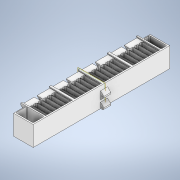
# Autodesk Inventor part: cajas_V2
Saved by Autodesk Inventor 2020.3 (Build 243373000, 373)
## iProperties
Created: 2021-02-18
Part Number: cajas_V2
Material: PET Plastic
Document SubType Name: Modeling
Designer: juanp
Density: 1.541 g/cm^3
Appearance: Polycarbonate - Clear
Author: juanp
Autodesk Inventor part; units mm, degrees
ref_plane "YZ Plane" through (0, 0, 0) normal (1, 0, 0) x (0, 1, 0)
ref_plane "XZ Plane" through (0, 0, 0) normal (0, 1, 0) x (-1, 0, 0)
ref_plane "XY Plane" through (0, 0, 0) normal (0, 0, 1) x (1, 0, 0)
sketch "Sketch1" plane through (0, 0, 0) normal (0, 1, 0) x (-1, 0, 0)
  line L0 (0, 0) -> (56, 0) construction
  line L1 (56, 0) -> (56, -330)
  line L2 (0, -330) -> (0, 0)
  line L3 (54, -4) -> (4, -4) construction
  line L4 (4, -4) -> (4, -15.1667)
  line L5 (4, -15.1667) -> (54, -15.1667)
  line L6 (54, -15.1667) -> (54, -4)
  line L7 (54, -19.1667) -> (4, -19.1667)
  line L8 (4, -19.1667) -> (4, -30.3333)
  line L9 (4, -30.3333) -> (54, -30.3333)
  line L10 (54, -30.3333) -> (54, -19.1667)
  line L11 (54, -32.3333) -> (4, -32.3333)
  line L12 (4, -32.3333) -> (4, -43.5)
  line L13 (4, -43.5) -> (54, -43.5)
  line L14 (54, -43.5) -> (54, -32.3333)
  line L15 (54, -45.5) -> (4, -45.5)
  line L16 (4, -45.5) -> (4, -56.6667)
  line L17 (4, -56.6667) -> (54, -56.6667)
  line L18 (54, -56.6667) -> (54, -45.5)
  line L19 (54, -58.6667) -> (4, -58.6667)
  line L20 (4, -58.6667) -> (4, -69.8333)
  line L21 (4, -69.8333) -> (54, -69.8333)
  line L22 (54, -69.8333) -> (54, -58.6667)
  line L23 (54, -71.8333) -> (4, -71.8333)
  line L24 (4, -71.8333) -> (4, -83)
  line L25 (4, -83) -> (54, -83)
  line L26 (54, -83) -> (54, -71.8333)
  line L27 (54, -85) -> (4, -85)
  line L28 (4, -85) -> (4, -96.1667)
  line L29 (4, -96.1667) -> (54, -96.1667)
  line L30 (54, -96.1667) -> (54, -85)
  line L31 (54, -102.1667) -> (4, -102.1667)
  line L32 (4, -102.1667) -> (4, -113.3333)
  line L33 (4, -113.3333) -> (54, -113.3333)
  line L34 (54, -113.3333) -> (54, -102.1667)
  line L35 (54, -115.3333) -> (4, -115.3333)
  line L36 (4, -115.3333) -> (4, -126.5)
  line L37 (4, -126.5) -> (54, -126.5)
  line L38 (54, -126.5) -> (54, -115.3333)
  line L39 (54, -128.5) -> (4, -128.5)
  line L40 (4, -128.5) -> (4, -139.6667)
  line L41 (4, -139.6667) -> (54, -139.6667)
  line L42 (54, -139.6667) -> (54, -128.5)
  line L43 (54, -141.6667) -> (4, -141.6667)
  line L44 (4, -141.6667) -> (4, -152.8333)
  line L45 (4, -152.8333) -> (54, -152.8333)
  line L46 (54, -152.8333) -> (54, -141.6667)
  line L47 (54, -154.8333) -> (4, -154.8333)
  line L48 (4, -154.8333) -> (4, -166)
  line L49 (4, -166) -> (54, -166)
  line L50 (54, -166) -> (54, -154.8333)
  line L51 (54, -168) -> (4, -168)
  line L52 (4, -168) -> (4, -179.1667)
  line L53 (4, -179.1667) -> (54, -179.1667)
  line L54 (54, -179.1667) -> (54, -168)
  line L55 (54, -185.1667) -> (4, -185.1667)
  line L56 (4, -185.1667) -> (4, -196.3333)
  line L57 (4, -196.3333) -> (54, -196.3333)
  line L58 (54, -196.3333) -> (54, -185.1667)
  line L59 (54, -198.3333) -> (4, -198.3333)
  line L60 (4, -198.3333) -> (4, -209.5)
  line L61 (4, -209.5) -> (54, -209.5)
  line L62 (54, -209.5) -> (54, -198.3333)
  line L63 (54, -211.5) -> (4, -211.5)
  line L64 (4, -211.5) -> (4, -222.6667)
  line L65 (4, -222.6667) -> (54, -222.6667)
  line L66 (54, -222.6667) -> (54, -211.5)
  line L67 (54, -224.6667) -> (4, -224.6667)
  line L68 (4, -224.6667) -> (4, -235.8333)
  line L69 (4, -235.8333) -> (54, -235.8333)
  line L70 (54, -235.8333) -> (54, -224.6667)
  line L71 (56, -330) -> (56, -349.1667)
  line L72 (56, -349.1667) -> (0, -349.1667) construction
  line L73 (0, -349.1667) -> (0, -330)
  line L74 (54, -237.8333) -> (4, -237.8333)
  line L75 (4, -237.8333) -> (4, -249)
  line L76 (4, -249) -> (54, -249)
  line L77 (54, -249) -> (54, -237.8333)
  line L78 (54, -251) -> (4, -251)
  line L79 (4, -251) -> (4, -262.1667)
  line L80 (4, -262.1667) -> (54, -262.1667)
  line L81 (54, -262.1667) -> (54, -251)
  line L82 (54, -268.1667) -> (4, -268.1667)
  line L83 (4, -268.1667) -> (4, -279.3333)
  line L84 (4, -279.3333) -> (54, -279.3333)
  line L85 (54, -279.3333) -> (54, -268.1667)
  line L86 (54, -281.3333) -> (4, -281.3333)
  line L87 (4, -281.3333) -> (4, -292.5)
  line L88 (4, -292.5) -> (54, -292.5)
  line L89 (54, -292.5) -> (54, -281.3333)
  line L90 (54, -294.5) -> (4, -294.5)
  line L91 (4, -294.5) -> (4, -305.6667)
  line L92 (4, -305.6667) -> (54, -305.6667)
  line L93 (54, -305.6667) -> (54, -294.5)
  line L94 (54, -307.6667) -> (4, -307.6667)
  line L95 (4, -307.6667) -> (4, -318.8333)
  line L96 (4, -318.8333) -> (54, -318.8333)
  line L97 (54, -318.8333) -> (54, -307.6667)
  line L98 (54, -320.8333) -> (4, -320.8333)
  line L99 (4, -320.8333) -> (4, -332)
  line L100 (4, -332) -> (54, -332)
  line L101 (54, -332) -> (54, -320.8333)
  line L102 (54, -334) -> (4, -334)
  line L103 (4, -334) -> (4, -345.1667)
  line L104 (4, -345.1667) -> (54, -345.1667)
  line L105 (54, -345.1667) -> (54, -334)
  line L106 (54, -4) -> (54, 16.4167)
  line L107 (54, 16.4167) -> (4, 16.4167)
  line L108 (4, 16.4167) -> (4, -4)
  line L109 (56, 0) -> (56, 20.4167)
  line L110 (56, 20.4167) -> (0, 20.4167)
  line L111 (0, 20.4167) -> (0, 0)
  line L112 (0, -349.1667) -> (0, -369.5833)
  line L113 (0, -369.5833) -> (56, -369.5833)
  line L114 (56, -369.5833) -> (56, -349.1667)
  line L115 (54, -339.5833) -> (104.9487, -339.5833) construction
  line L116 (104.9487, -339.5833) -> (104.9487, -9.5833) construction
  line L117 (104.9487, -9.5833) -> (54, -9.5833) construction
  line L118 (4, -349.1667) -> (54, -349.1667)
  line L119 (54, -349.1667) -> (54, -365.5833)
  line L120 (54, -365.5833) -> (4, -365.5833)
  line L121 (4, -365.5833) -> (4, -349.1667)
  point P0 (104.9487, -174.5833)
  dimension "d2" = 2
  dimension "d3" = 4
  dimension "d4" = 4
  dimension "d5" = 50
  dimension "d6" = 4
  dimension "d7" = 2
  dimension "d8" = 2
  dimension "d9" = 2
  dimension "d10" = 2
  dimension "d11" = 2
  dimension "d12" = 6
  dimension "d13" = 2
  dimension "d14" = 2
  dimension "d15" = 2
  dimension "d16" = 2
  dimension "d17" = 2
  dimension "d18" = 6
  dimension "d19" = 2
  dimension "d20" = 2
  dimension "d21" = 2
  dimension "d24" = 11.1667
  dimension "d35" = 2
  dimension "d36" = 2
  dimension "d37" = 6
  dimension "d38" = 2
  dimension "d39" = 2
  dimension "d40" = 2
  dimension "d41" = 2
  dimension "d42" = 2
  dimension "d59" = 4
  dimension "d60" = 330
  dimension "d212" = 4
  dimension "d332" = 195
  dimension "d333" = 195
  dimension "d334" = 4
  constraints: 244 end point, 53 parallel, 37 perpendicular, 34 equal length, 33 point on line, 28 horizontal, 8 collinear, 5 vertical, 3 midpoint
  measures "d2" distance between parallel lines of L1 L6
  measures "d3" distance between parallel lines of L0 L3
  measures "d4" distance between parallel lines of L4 L2
  measures "d5" distance of L3.start L3.end
  measures "d6" distance between parallel lines of L7 L5
  measures "d7" distance between parallel lines of L11 L9
  measures "d8" distance between parallel lines of L15 L13
  measures "d9" distance between parallel lines of L19 L17
  measures "d10" distance between parallel lines of L21 L23
  measures "d11" distance between parallel lines of L27 L25
  measures "d12" distance between parallel lines of L31 L29
  measures "d13" distance between parallel lines of L35 L33
  measures "d14" distance between parallel lines of L39 L37
  measures "d15" distance between parallel lines of L43 L41
  measures "d16" distance between parallel lines of L47 L45
  measures "d17" distance between parallel lines of L51 L49
  measures "d18" distance between parallel lines of L55 L53
  measures "d19" distance between parallel lines of L59 L57
  measures "d20" distance between parallel lines of L63 L61
  measures "d21" distance between parallel lines of L67 L65
  measures "d24" distance of L61.end L59.start
  measures "d35" distance between parallel lines of L69 L74
  measures "d36" distance between parallel lines of L78 L76
  measures "d37" distance between parallel lines of L82 L80
  measures "d38" distance between parallel lines of L86 L84
  measures "d39" distance between parallel lines of L90 L88
  measures "d40" distance between parallel lines of L94 L92
  measures "d41" distance between parallel lines of L98 L96
  measures "d42" distance between parallel lines of L102 L100
  measures "d59" distance between parallel lines of L72 L104
  measures "d60" distance of L117.end L115.start
  measures "d212" distance between parallel lines of L107 L110
  measures "d332" distance from line of L110 point (104.949, -174.583)
  measures "d333" distance from line of L113 point (104.949, -174.583)
  measures "d334" distance between parallel lines of L113 L120
extrude "Extrusion1" add sketch "Sketch1" along normal blind 50
sketch "Sketch3" plane through (0, 0, 0) normal (0, -1, 0) x (1, 0, 0)
  line L0 (-56, -369.5833) -> (-56, 20.4167) projected
  line L1 (0, 20.4167) -> (0, -369.5833) projected
  line L2 (-56, 20.4167) -> (0, 20.4167) projected
  line L3 (0, -369.5833) -> (-56, -369.5833) projected
extrude "Extrusion3" add sketch "Sketch3" along normal blind 2
chamfer "Chamfer4" distance 2 angle 45 208 edges at (-54, 25, -128.5) (-4, 25, -126.5) (-54, 25, -141.6667) (-54, 25, -179.1667) (-54, 25, -185.1667) (-4, 25, -141.6667) (-4, 25, -139.6667) (-54, 25, -115.3333) (-4, 25, -115.3333) (-4, 25, -345.1667) (-54, 25, -345.1667) (-4, 25, -128.5) (-4, 25, -332) (-4, 25, -334) (-54, 25, -334) (-54, 25, -332) (-4, 25, -320.8333) (-54, 25, -318.8333) (-4, 25, -318.8333) (-54, 25, -320.8333) (-4, 25, -307.6667) (-54, 25, -305.6667) (-54, 25, -307.6667) (-4, 25, -305.6667) (-4, 25, -294.5) (-54, 25, -292.5) (-4, 25, -292.5) (-54, 25, -294.5) (-4, 25, -281.3333) (-4, 25, -268.1667) (-54, 25, -279.3333) (-4, 25, -279.3333) (-54, 25, -281.3333) (-4, 25, -166) (-4, 25, -168) (-4, 25, -179.1667) (-4, 25, -196.3333) (-4, 25, -185.1667) (-4, 25, -209.5) (-4, 25, -198.3333) (-54, 0, -173.5833) (-4, 0, -173.5833) (-29, 0, -179.1667) (-29, 0, -185.1667) (-54, 0, -190.75) (-4, 0, -190.75) (-4, 0, -203.9167) (-29, 0, -198.3333) (-54, 0, -203.9167) (-29, 0, -196.3333) (-54, 0, -217.0833) (-4, 0, -217.0833) (-29, 0, -222.6667) (-29, 0, -209.5) (-54, 25, -196.3333) (-54, 25, -198.3333) (-54, 25, -209.5) (-4, 25, -211.5) (-54, 25, -211.5) (-54, 25, -222.6667) (-4, 25, -222.6667) (-4, 25, -224.6667) (-54, 25, -224.6667) (-4, 25, -251) (-54, 25, -249) (-4, 25, -249) (-54, 25, -251) (-4, 25, -262.1667) (-54, 25, -262.1667) (-54, 25, -268.1667) (-29, 0, -211.5) (-29, 0, -224.6667) (-54, 0, -230.25) (-4, 0, -230.25) (-29, 0, -235.8333) (-29, 0, -237.8333) (-54, 0, -243.4167) (-4, 0, -243.4167) (-29, 0, -249) (-29, 0, -251) (-54, 0, -256.5833) (-29, 0, -262.1667) (-29, 0, -268.1667) (-54, 0, -273.75) (-29, 0, -279.3333) (-4, 0, -273.75) (-54, 0, -286.9167) (-29, 0, -292.5) (-4, 0, -256.5833) (-29, 0, -281.3333) (-4, 0, -286.9167) (-29, 0, -294.5) (-54, 0, -300.0833) (-4, 0, -300.0833) (-29, 0, -305.6667) (-29, 0, -307.6667) (-54, 0, -313.25) (-4, 0, -313.25) (-29, 0, -318.8333) (-29, 0, -320.8333) (-29, 0, -332) (-4, 0, -326.4167) (-29, 0, -334) (-4, 0, -339.5833) (-29, 0, -345.1667) (-54, 0, -339.5833) (-54, 0, -326.4167) (-4, 25, -237.8333) (-4, 25, -235.8333) (-54, 25, -235.8333) (-54, 25, -237.8333) (-54, 25, -126.5) (-54, 25, -113.3333) (-4, 25, -113.3333) (-4, 25, -102.1667) (-54, 25, -102.1667) (-54, 25, -96.1667) (-4, 25, -96.1667) (-4, 25, -85) (-54, 25, -85) (-29, 0, -96.1667) (-4, 0, -90.5833) (-29, 0, -85) (-29, 0, -83) (-4, 0, -77.4167) (-29, 0, -71.8333) (-54, 0, -77.4167) (-54, 0, -90.5833) (-54, 25, -83) (-4, 25, -83) (-4, 25, -71.8333) (-54, 25, -71.8333) (-54, 25, -69.8333) (-4, 25, -69.8333) (-4, 25, -58.6667) (-54, 25, -58.6667) (-54, 25, -56.6667) (-54, 25, -45.5) (-54, 25, -43.5) (-4, 25, -56.6667) (-54, 25, -32.3333) (-4, 25, -43.5) (-54, 25, -30.3333) (-4, 25, -32.3333) (-4, 25, -30.3333) (-54, 25, -19.1667) (-4, 25, -19.1667) (-4, 25, -45.5) (-54, 0, -24.75) (-54, 25, -15.1667) (-4, 25, -15.1667) (-29, 0, -43.5) (-29, 0, -32.3333) (-4, 0, -37.9167) (-29, 0, -30.3333) (-4, 0, -24.75) (-29, 0, -19.1667) (-54, 0, -37.9167) (-29, 0, -69.8333) (-54, 0, -64.25) (-4, 0, -64.25) (-29, 0, -58.6667) (-29, 0, -56.6667) (-4, 0, -51.0833) (-29, 0, -45.5) (-54, 0, -51.0833) (-4, 25, -154.8333) (-4, 25, -152.8333) (-54, 25, -152.8333) (-54, 25, -139.6667) (-29, 0, -168) (-29, 0, -166) (-29, 0, -154.8333) (-4, 0, -160.4167) (-29, 0, -152.8333) (-4, 0, -147.25) (-29, 0, -141.6667) (-4, 0, -134.0833) (-29, 0, -128.5) (-54, 0, -147.25) (-54, 0, -160.4167) (-29, 0, -102.1667) (-54, 0, -107.75) (-4, 0, -107.75) (-29, 0, -113.3333) (-29, 0, -115.3333) (-29, 0, -126.5) (-4, 0, -120.9167) (-29, 0, -139.6667) (-54, 0, -134.0833) (-54, 0, -120.9167) (-54, 25, -154.8333) (-54, 25, -166) (-54, 25, -168) (-4, 25, 16.4167) (-54, 25, 16.4167) (-29, 0, 16.4167) (-54, 0, 0.625) (-29, 0, -15.1667) (-4, 0, 0.625) (-29, 0, -365.5833) (-4, 0, -357.375) (-4, 25, -365.5833) (-54, 25, -349.1667) (-54, 0, -357.375) (-29, 0, -349.1667) (-4, 25, -349.1667) (-54, 25, -365.5833)
ref_plane "Plano medio efectivo" through (-6, 2, -174.5833) normal (0, 0, -1) x (-1, 0, 0)
sketch "Sketch57" plane through (-6, 50, -349.1667) normal (0, 0, -1) x (-1, 0, 0)
  line L0 (50, -52) -> (50, 0) projected
  line L1 (50, 0) -> (65, 0)
  line L2 (65, 0) -> (50, -15)
  point P0 (-6, -50)
  dimension "d335" = 45
  dimension "d336" = 15
  constraints: 4 end point, 1 horizontal, 1 point on line
  measures "d335" angle of L0 L2
  measures "d336" distance of L0.end L1.end
extrude "Extrusion46" add sketch "Sketch57" against normal up to surface (334 mm away)
sketch "Sketch58" plane through (0, 50, 0) normal (0, 1, 0) x (1, 0, 0)
  line L0 (0, -20.4167) -> (0, 369.5833) projected
  line L1 (-71, 349.1667) -> (-71, 15.1667) projected
  line L2 (-71, 349.1667) -> (-56, 349.1667) projected
  line L3 (-71, 349.1667) -> (0, 349.1667)
  line L4 (-71, 15.1667) -> (0, 15.1667)
  line L5 (-2, 349.1667) -> (-2, 15.1667)
  line L6 (-4, 28.3333) -> (-4, 21.1667) projected
  line L7 (-4, 24.75) -> (0, 24.75) construction
  line L8 (-6, 19.1667) -> (-52, 19.1667) projected
  line L9 (-29, 19.1667) -> (-29, 15.1667) construction
  line L10 (-52, 15.1667) -> (-6, 15.1667) projected
  line L11 (-6, 102.1667) -> (-52, 102.1667) projected
  line L12 (-29, 102.1667) -> (-29, 100.1667) construction
  line L13 (-29, 100.1667) -> (-29, 98.1667) construction
  line L14 (-29, 98.1667) -> (-29, 96.1667) construction
  line L15 (-6, 96.1667) -> (-52, 96.1667) projected
  line L16 (-6, 179.1667) -> (-52, 179.1667) projected
  line L17 (-29, 179.1667) -> (-29, 181.1667) construction
  line L18 (-29, 181.1667) -> (-29, 183.1667) construction
  line L19 (-29, 183.1667) -> (-29, 185.1667) construction
  line L20 (-6, 185.1667) -> (-52, 185.1667) projected
  line L21 (-52, 262.1667) -> (-6, 262.1667) projected
  line L22 (-29, 262.1667) -> (-29, 264.1667) construction
  line L23 (-29, 264.1667) -> (-29, 266.1667) construction
  line L24 (-29, 266.1667) -> (-29, 268.1667) construction
  line L25 (-6, 268.1667) -> (-52, 268.1667) projected
  line L26 (-6, 345.1667) -> (-52, 345.1667) projected
  line L27 (-6, 349.1667) -> (-52, 349.1667) projected
  line L28 (-29, 349.1667) -> (-29, 345.1667) construction
  line L29 (-2, 347.1667) -> (-71, 347.1667)
  line L30 (-71, 266.1667) -> (-2, 266.1667)
  line L31 (-71, 264.1667) -> (-2, 264.1667)
  line L32 (-2, 183.1667) -> (-71, 183.1667)
  line L33 (-71, 181.1667) -> (-2, 181.1667)
  line L34 (-71, 98.1667) -> (-2, 98.1667)
  line L35 (-2, 100.1667) -> (-71, 100.1667)
  line L36 (-2, 17.1667) -> (-71, 17.1667)
  point P0 (-2, 24.75)
  point P1 (-29, 347.1667)
  point P2 (-29, 17.1667)
  constraints: 44 end point, 17 point on line, 14 midpoint, 9 horizontal, 6 collinear, 3 perpendicular, 2 vertical, 21 other
extrude "Extrusion47" add sketch "Sketch58" along normal blind 3 contours L4 L5 L3 L0 | L4 L1 L36 L5 | L5 L29 L1 L2 L3 | L34 L1 L35 L5 | L5 L31 L1 L30 | L33 L1 L32 L5
sketch "Sketch59" plane through (0, 53, 0) normal (0, 1, 0) x (1, 0, 0)
  line L0 (-2, 266.1667) -> (-71, 266.1667) projected
  line L1 (-71, 266.1667) -> (-71, 264.1667) projected
  line L2 (-71, 264.1667) -> (-2, 264.1667) projected
  line L3 (-2, 264.1667) -> (-2, 183.1667) projected
  line L4 (-2, 183.1667) -> (-71, 183.1667) projected
  line L5 (-71, 183.1667) -> (-71, 181.1667) projected
  line L6 (-71, 181.1667) -> (-2, 181.1667) projected
  line L7 (-2, 181.1667) -> (-2, 100.1667) projected
  line L8 (-2, 100.1667) -> (-71, 100.1667) projected
  line L9 (-71, 100.1667) -> (-71, 98.1667) projected
  line L10 (-71, 98.1667) -> (-2, 98.1667) projected
  line L11 (-2, 98.1667) -> (-2, 17.1667) projected
  line L12 (-2, 17.1667) -> (-71, 17.1667) projected
  line L13 (-71, 17.1667) -> (-71, 15.1667) projected
  line L14 (-71, 15.1667) -> (0, 15.1667) projected
  line L15 (0, 15.1667) -> (0, 349.1667) projected
  line L16 (0, 349.1667) -> (-71, 349.1667) projected
  line L17 (-71, 349.1667) -> (-71, 347.1667) projected
  line L18 (-71, 347.1667) -> (-2, 347.1667) projected
  line L19 (-2, 347.1667) -> (-2, 266.1667) projected
  line L20 (-71, 98.1667) -> (-71, 17.1667) projected
  line L21 (-71, 181.1667) -> (-71, 100.1667) projected
  line L22 (-71, 264.1667) -> (-71, 183.1667) projected
  line L23 (-71, 347.1667) -> (-71, 266.1667) projected
  line L24 (-71, 345.1667) -> (-3.8049, 345.1667)
  line L25 (-3.8049, 345.1667) -> (-3.8049, 268.1667)
  line L26 (-3.8049, 268.1667) -> (-71, 268.1667)
  line L27 (-71, 268.1667) -> (-71, 345.1667)
  line L28 (-71, 262.1667) -> (-4, 262.1667)
  line L29 (-4, 262.1667) -> (-4, 185.1667)
  line L30 (-4, 185.1667) -> (-71, 185.1667)
  line L31 (-71, 185.1667) -> (-71, 262.1667)
  line L32 (-71, 179.1667) -> (-4, 179.1667)
  line L33 (-4, 179.1667) -> (-4, 102.1667)
  line L34 (-4, 102.1667) -> (-71, 102.1667)
  line L35 (-71, 102.1667) -> (-71, 179.1667)
  line L36 (-71, 96.1667) -> (-4, 96.1667)
  line L37 (-4, 96.1667) -> (-4, 19.1667)
  line L38 (-4, 19.1667) -> (-71, 19.1667)
  line L39 (-71, 19.1667) -> (-71, 96.1667)
  point P0 (0, 0)
  dimension "d341" = 2
  dimension "d342" = 1.8049
  dimension "d343" = 2
  dimension "d344" = 2
  dimension "d345" = 2
  dimension "d346" = 2
  dimension "d347" = 2
  dimension "d348" = 2
  dimension "d349" = 2
  dimension "d350" = 2
  dimension "d351" = 2
  constraints: 32 end point, 8 parallel, 5 point on line, 4 horizontal, 4 perpendicular
  measures "d341" distance between parallel lines of L18 L24
  measures "d342" distance between parallel lines of L19 L25
  measures "d343" distance between parallel lines of L0 L26
  measures "d344" distance between parallel lines of L28 L2
  measures "d345" distance between parallel lines of L4 L30
  measures "d346" distance between parallel lines of L32 L6
  measures "d347" distance between parallel lines of L8 L34
  measures "d348" distance between parallel lines of L36 L10
  measures "d349" distance between parallel lines of L12 L38
  measures "d350" distance between parallel lines of L3 L29
  measures "d351" distance between parallel lines of L7 L33
extrude "Extrusion48" add sketch "Sketch59" along normal blind 2 contours L19 L18 L17 L16 L15 L14 L13 L12 L11 L10 L9 L8 L7 L6 L5 L4 L3 L2 L1 L0 | L0 L23 L26 L25 L24 L18 L19 | L2 L3 L4 L22 L30 L29 L28 | L6 L7 L8 L21 L34 L33 L32 | L20 L38 L37 L36 L10 L11 L12
chamfer "Chamfer11" distance 1.999 angle 45 12 edges at (-36.5, 53, -17.1667) (-2, 53, -57.6667) (-2, 53, -140.6667) (-36.5, 53, -98.1667) (-36.5, 53, -100.1667) (-36.5, 53, -181.1667) (-36.5, 53, -183.1667) (-2, 53, -223.6667) (-36.5, 53, -264.1667) (-36.5, 53, -266.1667) (-2, 53, -306.6667) (-36.5, 53, -347.1667)
sketch "Sketch60" plane through (0, 50, 0) normal (0, 1, 0) x (1, 0, 0)
  line L0 (-52, 15.1667) -> (-56, 15.1667) projected
  line L1 (-56, 15.1667) -> (-56, -20.4167) projected
  line L2 (-56, -20.4167) -> (0, -20.4167) projected
  line L3 (0, -20.4167) -> (0, 15.1667) projected
  line L4 (0, 15.1667) -> (-6, 15.1667) projected
  line L5 (-4, 13.1667) -> (-6, 15.1667) projected
  line L6 (-4, 13.1667) -> (-4, -14.4167) projected
  line L7 (-6, -16.4167) -> (-4, -14.4167) projected
  line L8 (-6, -16.4167) -> (-52, -16.4167) projected
  line L9 (-54, -14.4167) -> (-52, -16.4167) projected
  line L10 (-54, -14.4167) -> (-54, 13.1667) projected
  line L11 (-52, 15.1667) -> (-54, 13.1667) projected
  line L12 (-6, 349.1667) -> (0, 349.1667) projected
  line L13 (0, 349.1667) -> (0, 369.5833) projected
  line L14 (0, 369.5833) -> (-56, 369.5833) projected
  line L15 (-56, 369.5833) -> (-56, 349.1667) projected
  line L16 (-56, 349.1667) -> (-52, 349.1667) projected
  line L17 (-54, 351.1667) -> (-52, 349.1667) projected
  line L18 (-54, 351.1667) -> (-54, 363.5833) projected
  line L19 (-52, 365.5833) -> (-54, 363.5833) projected
  line L20 (-52, 365.5833) -> (-6, 365.5833) projected
  line L21 (-4, 363.5833) -> (-6, 365.5833) projected
  line L22 (-4, 363.5833) -> (-4, 351.1667) projected
  line L23 (-6, 349.1667) -> (-4, 351.1667) projected
  point P0 (0, 0)
extrude "Extrusion49" add sketch "Sketch60" along normal up to surface (5 mm away)
sketch "Sketch61" plane through (0, 50, 0) normal (0, 1, 0) x (1, 0, 0)
  line L0 (-56, -20.4167) -> (-56, 369.5833) projected
  line L1 (-56, 15.1667) -> (-56, 349.1667) projected
  line L2 (-71, 347.1667) -> (-71, 266.1667) projected
  line L3 (-56, 310.4167) -> (-71, 310.4167)
  line L4 (-71, 310.4167) -> (-71, 302.9167)
  line L5 (-71, 302.9167) -> (-56, 302.9167)
  line L6 (-56, 302.9167) -> (-56, 310.4167)
  line L7 (-56, 227.4167) -> (-71, 227.4167)
  line L8 (-71, 227.4167) -> (-71, 219.9167)
  line L9 (-71, 219.9167) -> (-56, 219.9167)
  line L10 (-56, 219.9167) -> (-56, 227.4167)
  line L11 (-56, 144.4167) -> (-71, 144.4167)
  line L12 (-71, 144.4167) -> (-71, 136.9167)
  line L13 (-71, 136.9167) -> (-56, 136.9167)
  line L14 (-56, 136.9167) -> (-56, 144.4167)
  line L15 (-56, 61.4167) -> (-71, 61.4167)
  line L16 (-71, 61.4167) -> (-71, 53.9167)
  line L17 (-71, 53.9167) -> (-56, 53.9167)
  line L18 (-56, 53.9167) -> (-56, 61.4167)
  point P0 (0, 0)
  point P1 (-71, 306.6667)
  point P2 (-71, 223.6667)
  point P3 (-71, 140.6667)
  point P4 (-71, 57.6667)
  dimension "d359" = 7.5
  dimension "d362" = 83
  constraints: 32 end point, 2 midpoint, 2 parallel, 2 point on line, 1 horizontal, 1 perpendicular, 1 vertical, 27 other
  measures "d359" distance between parallel lines of L5 L3
  measures "d362" distance of L3.start L7.start
extrude "Extrusion50" cut sketch "Sketch61" against normal up to next
ref_plane "Work Plane14" through (-56, 50, -297.5167) normal (0, 0, -1) x (-1, 0, 0)
sketch "Sketch62" plane through (-56, 50, -297.5167) normal (0, 0, -1) x (-1, 0, 0)
  line L0 (0, -15) -> (15, 0) projected
  line L1 (0, -52) -> (0, 5) projected
  line L2 (0, -50.233) -> (10, -40.233)
  line L3 (0, -50.233) -> (14.1421, -50.233) construction
  line L4 (10, -40.233) -> (10, -5)
  line L5 (10, -40.233) -> (0, -40.233) construction
  line L6 (5, -40.233) -> (5, -34.183) construction
  line L7 (5, -34.183) -> (5, -19.183) construction
  circle A0 centre (5, -34.183) radius 1.65
  circle A1 centre (5, -19.183) radius 1.65
  point P0 (-56, -50)
  dimension "d387" = 45
  dimension "d388" = 6.05
  dimension "d389" = 15
  dimension "d390" = 5
  dimension "d391" = 11.767
  dimension "d392" = 3.3
  constraints: 12 end point, 4 point on line, 2 centre point, 2 coincident, 2 horizontal, 2 vertical, 1 equal length, 1 equal radius, 1 midpoint
  measures "d387" angle of L3 L2
  measures "d388" distance of L6.start L6.end
  measures "d389" distance of L6.end L7.end
  measures "d390" distance between parallel lines of L1 L6
  measures "d391" distance from line of L5 L1.start
  measures "d392" diameter of A0
extrude "Extrusion51" add sketch "Sketch62" against normal blind 5
sketch "Sketch63" plane through (-56, 50, -297.5167) normal (0, 0, -1) x (-1, 0, 0)
  circle A0 centre (5, -19.183) radius 1.65 projected
  line L0 (3.4123, -16.433) -> (6.5877, -16.433)
  line L1 (6.5877, -16.433) -> (8.1754, -19.183)
  line L2 (8.1754, -19.183) -> (6.5877, -21.933)
  line L3 (6.5877, -21.933) -> (3.4123, -21.933)
  line L4 (3.4123, -21.933) -> (1.8246, -19.183)
  line L5 (1.8246, -19.183) -> (3.4123, -16.433)
  circle A1 centre (5, -34.183) radius 1.65 projected
  line L6 (3.4123, -31.433) -> (6.5877, -31.433)
  line L7 (6.5877, -31.433) -> (8.1754, -34.183)
  line L8 (8.1754, -34.183) -> (6.5877, -36.933)
  line L9 (6.5877, -36.933) -> (3.4123, -36.933)
  line L10 (3.4123, -36.933) -> (1.8246, -34.183)
  line L11 (1.8246, -34.183) -> (3.4123, -31.433)
  point P0 (-56, -50)
  dimension "d398" = 5.5
  constraints: 24 end point, 2 coincident, 2 horizontal, 1 parallel, 26 other
  measures "d398" distance between parallel lines of L0 L3
extrude "Extrusion52" cut sketch "Sketch63" against normal blind 2.5
pattern_linear "Rectangular Pattern9" count 4 spacing 83 along (0, 0, 1) of "Extrusion51", "Extrusion52"
ref_plane "Plano de corte" through (-6, 50, -182.1667) normal (0, 0, -1) x (-1, 0, 0)
sketch "Sketch65" plane through (-6, 50, -182.1667) normal (0, 0, -1) x (-1, 0, 0)
  line L0 (-15.3, -45.4239) -> (-12.5761, -42.7)
  line L1 (-12.5761, -42.7) -> (-8.7239, -42.7) construction
  line L2 (-8.7239, -42.7) -> (-6, -45.4239) construction
  line L3 (-6, -45.4239) -> (-6, -49.2761) construction
  line L4 (-6, -49.2761) -> (-8.7239, -52) construction
  line L5 (-8.7239, -52) -> (-12.5761, -52)
  line L6 (-12.5761, -52) -> (-15.3, -49.2761)
  line L7 (-15.3, -49.2761) -> (-15.3, -45.4239)
  line L8 (-6, -17.2569) -> (-6, -21.1091) construction
  line L9 (-6, -21.1091) -> (-8.7239, -23.833) construction
  line L10 (-8.7239, -23.833) -> (-12.5761, -23.833) construction
  line L11 (-12.5761, -23.833) -> (-15.3, -21.1091)
  line L12 (-15.3, -21.1091) -> (-15.3, -17.2569)
  line L13 (-15.3, -17.2569) -> (-12.5761, -14.533)
  line L14 (-12.5761, -14.533) -> (-8.7239, -14.533) construction
  line L15 (-8.7239, -14.533) -> (-6, -17.2569) construction
  line L16 (50.35, -17.2569) -> (53.0739, -14.533) construction
  line L17 (53.0739, -14.533) -> (56.9261, -14.533) construction
  line L18 (56.9261, -14.533) -> (59.65, -17.2569)
  line L19 (59.65, -17.2569) -> (59.65, -21.1091)
  line L20 (59.65, -21.1091) -> (56.9261, -23.833)
  line L21 (56.9261, -23.833) -> (53.0739, -23.833) construction
  line L22 (53.0739, -23.833) -> (50.35, -21.1091) construction
  line L23 (50.35, -21.1091) -> (50.35, -17.2569) construction
  line L24 (59.65, -49.2761) -> (56.9261, -52)
  line L25 (56.9261, -52) -> (53.0739, -52)
  line L26 (53.0739, -52) -> (50.35, -49.2761) construction
  line L27 (50.35, -49.2761) -> (50.35, -45.4239) construction
  line L28 (50.35, -45.4239) -> (53.0739, -42.7) construction
  line L29 (53.0739, -42.7) -> (56.9261, -42.7) construction
  line L30 (56.9261, -42.7) -> (59.65, -45.4239)
  line L31 (59.65, -45.4239) -> (59.65, -49.2761)
  line L32 (-10.65, -19.183) -> (55, -19.183) construction
  line L33 (55, -19.183) -> (55, -47.35) construction
  line L34 (55, -47.35) -> (-10.65, -47.35) construction
  line L35 (-10.65, -47.35) -> (-10.65, -19.183) construction
  line L36 (-10.65, -19.183) -> (55, -47.35) construction
  line L37 (55, -19.183) -> (-10.65, -47.35) construction
  circle A0 centre (-10.65, -19.183) radius 1.65
  circle A1 centre (-10.65, -47.35) radius 1.65
  circle A2 centre (55, -47.35) radius 1.65
  circle A3 centre (55, -19.183) radius 1.65
  line L38 (-6, -52) -> (50, -52) projected
  circle A4 centre (55, -19.183) radius 1.65 projected
  line L39 (-6, 5) -> (-6, -52) projected
  line L40 (-12.5761, -14.533) -> (-6, -7.9569)
  line L41 (-12.5761, -23.833) -> (-6, -30.4091)
  line L42 (-12.5761, -42.7) -> (-6, -36.1239)
  line L43 (-8.7239, -52) -> (-6, -52)
  line L44 (50, -52) -> (53.0739, -52)
  line L45 (56.9261, -42.7) -> (50, -35.7739)
  line L46 (50, -50.233) -> (50, -15) projected
  line L47 (50, -30.7591) -> (56.9261, -23.833)
  line L48 (56.9261, -14.533) -> (53.6965, -11.3035)
  line L49 (50, -15) -> (65, 0) projected
  line L50 (50, -52) -> (50, 5) projected
  point P0 (22.175, -33.2665)
  dimension "d403" = 3
  constraints: 92 end point, 8 coincident, 8 collinear, 6 horizontal, 6 parallel, 6 point on line, 4 centre point, 4 equal radius, 2 midpoint, 1 concentric, 1 perpendicular, 68 other
  measures "d403" distance edge to line of A2 L31
extrude "Extrusion53" add sketch "Sketch65" along normal mid plane 20
sketch "Sketch66" plane through (-6, 50, -192.1667) normal (0, 0, -1) x (-1, 0, 0)
  circle A0 centre (-10.65, -19.183) radius 1.65 projected
  circle A1 centre (-10.65, -47.35) radius 1.65 projected
  circle A2 centre (55, -47.35) radius 1.65 projected
  circle A3 centre (55, -19.183) radius 1.65 projected
  line L0 (-9.0623, -21.933) -> (-12.2377, -21.933)
  line L1 (-12.2377, -21.933) -> (-13.8254, -19.183)
  line L2 (-13.8254, -19.183) -> (-12.2377, -16.433)
  line L3 (-12.2377, -16.433) -> (-9.0623, -16.433)
  line L4 (-9.0623, -16.433) -> (-7.4746, -19.183)
  line L5 (-7.4746, -19.183) -> (-9.0623, -21.933)
  line L6 (-13.8254, -47.35) -> (-12.2377, -44.6)
  line L7 (-12.2377, -44.6) -> (-9.0623, -44.6)
  line L8 (-9.0623, -44.6) -> (-7.4746, -47.35)
  line L9 (-7.4746, -47.35) -> (-9.0623, -50.1)
  line L10 (-9.0623, -50.1) -> (-12.2377, -50.1)
  line L11 (-12.2377, -50.1) -> (-13.8254, -47.35)
  line L12 (51.8246, -47.35) -> (53.4123, -44.6)
  line L13 (53.4123, -44.6) -> (56.5877, -44.6)
  line L14 (56.5877, -44.6) -> (58.1754, -47.35)
  line L15 (58.1754, -47.35) -> (56.5877, -50.1)
  line L16 (56.5877, -50.1) -> (53.4123, -50.1)
  line L17 (53.4123, -50.1) -> (51.8246, -47.35)
  circle A4 centre (55, -19.183) radius 1.65 projected
  line L18 (53.4123, -16.433) -> (56.5877, -16.433)
  line L19 (56.5877, -16.433) -> (58.1754, -19.183)
  line L20 (58.1754, -19.183) -> (56.5877, -21.933)
  line L21 (56.5877, -21.933) -> (53.4123, -21.933)
  line L22 (53.4123, -21.933) -> (51.8246, -19.183)
  line L23 (51.8246, -19.183) -> (53.4123, -16.433)
  point P0 (-6, -50)
  dimension "d406" = 5.5
  constraints: 48 end point, 4 coincident, 4 horizontal, 3 equal length, 52 other
  measures "d406" distance between parallel lines of L3 L0
extrude "Extrusion54" cut sketch "Sketch66" against normal blind 2.5
chamfer "Chamfer12" distance 0.6667 angle 45 48 edges at (-29, 50, -345.1667) (-29, 50, -334) (-29, 50, -332) (-29, 50, -320.8333) (-29, 50, -318.8333) (-29, 50, -307.6667) (-29, 50, -305.6667) (-29, 50, -294.5) (-29, 50, -292.5) (-29, 50, -281.3333) (-29, 50, -279.3333) (-29, 50, -262.1667) (-29, 50, -251) (-29, 50, -249) (-29, 50, -237.8333) (-29, 50, -235.8333) (-29, 50, -224.6667) (-29, 50, -222.6667) (-29, 50, -209.5) (-29, 50, -211.5) (-29, 50, -198.3333) (-29, 50, -196.3333) (-29, 50, -179.1667) (-29, 50, -168) (-29, 50, -166) (-29, 50, -154.8333) (-29, 50, -152.8333) (-29, 50, -141.6667) (-29, 50, -139.6667) (-29, 50, -128.5) (-29, 50, -126.5) (-29, 50, -115.3333) (-29, 50, -113.3333) (-29, 50, -96.1667) (-29, 50, -85) (-29, 50, -83) (-29, 50, -71.8333) (-29, 50, -69.8333) (-29, 50, -58.6667) (-29, 50, -56.6667) (-29, 50, -43.5) (-29, 50, -45.5) (-29, 50, -32.3333) (-29, 50, -30.3333) (-29, 50, -19.1667) (-29, 50, -102.1667) (-29, 50, -185.1667) (-29, 50, -268.1667)
equation "\"d2\" = grosor_pared"
equation "\"d5\" = largo_cajas"
equation "\"d7\" = grosor_pared"
equation "\"d8\" = grosor_pared"
equation "\"d10\" = grosor_pared"
equation "\"d14\" = grosor_pared"
equation "\"d15\" = grosor_pared"
equation "\"d16\" = grosor_pared"
equation "\"d19\" = grosor_pared"
equation "\"d20\" = grosor_pared"
equation "\"d21\" = grosor_pared"
equation "\"d25\" = altura_cajas"
equation "\"d32\" = grosor_pared"
equation "\"largo_cajas\" = 50"
equation "\"grosor_pared\" = 2"
equation "\"altura_cajas\" = 50"
body "Solid1"
